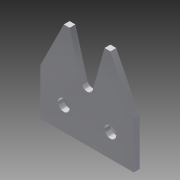
# Autodesk Inventor part: pickup arm tab
Saved by Autodesk Inventor 2015 (Build 190159000, 159)
## iProperties
Created: 2015-01-20
Part Number: pickup arm tab
Material: Aluminum 6061
Document SubType Name: Modeling
Designer: Jarod
Density: 2.7 g/cm^3
Appearance: Aluminum - Flat
Author: Jarod
Autodesk Inventor part; units mm, degrees
ref_plane "YZ Plane" through (0, 0, 0) normal (1, 0, 0) x (0, 1, 0)
ref_plane "XZ Plane" through (0, 0, 0) normal (0, 1, 0) x (-1, 0, 0)
ref_plane "XY Plane" through (0, 0, 0) normal (0, 0, 1) x (1, 0, 0)
sketch "Sketch1" plane through (0, 0, 0) normal (0, 0, 1) x (1, 0, 0)
  line L0 (0, 0) -> (50.8, 0)
  line L1 (50.8, 0) -> (50.8, 50.8)
  line L2 (50.8, 50.8) -> (0, 50.8)
  line L3 (0, 50.8) -> (0, 0)
  dimension "d0" = 50.8
  dimension "d1" = 50.8
  constraints: 8 end point, 2 parallel, 1 horizontal, 1 perpendicular
  measures "d0" distance of L2.end L1.end
  measures "d1" distance of L1.end L0.end
extrude "Extrusion1" add sketch "Sketch1" along normal blind 3.175
sketch "Sketch2" plane through (0, 0, 3.175) normal (0, 0, 1) x (1, 0, 0)
  line L0 (0, 0) -> (50.8, 0) projected
  line L1 (50.8, 0) -> (50.8, 50.8) projected
  line L2 (50.8, 50.8) -> (0, 50.8) projected
  line L3 (0, 50.8) -> (0, 0) projected
  point P0 (12.7, 12.7)
  point P1 (38.1, 12.7)
  dimension "d4" = 12.7
  dimension "d5" = 12.7
  dimension "d6" = 12.7
  dimension "d7" = 12.7
  measures "d4" distance from line of L0 point (12.7, 12.7)
  measures "d5" distance from line of L3 point (12.7, 12.7)
  measures "d6" distance from line of L0 point (38.1, 12.7)
  measures "d7" distance from line of L1 point (38.1, 12.7)
hole "Hole1" at (12.7, 12.7, 3.175) at (38.1, 12.7, 3.175) direction (0, 0, -1) diameter 6.35 end through all
sketch "Sketch3" plane through (0, 0, 0) normal (0, 0, -1) x (-1, 0, 0)
  line L0 (0, 0) -> (-50.8, 0) projected
  line L1 (-50.8, 0) -> (-50.8, 50.8) projected
  line L2 (-50.8, 0) -> (-50.8, 50.8) projected
  line L3 (-50.8, 25.4) -> (-38.1, 50.8)
  line L4 (-50.8, 50.8) -> (0, 50.8) construction
  line L5 (-38.1, 50.8) -> (-12.7, 50.8) construction
  line L6 (-12.7, 50.8) -> (0, 25.4)
  line L7 (0, 50.8) -> (0, 0) projected
  line L8 (-38.1, 50.8) -> (-50.8, 50.8)
  line L9 (-50.8, 50.8) -> (-50.8, 25.4)
  line L10 (-12.7, 50.8) -> (0, 50.8)
  line L11 (0, 50.8) -> (0, 25.4)
  dimension "d19" = 25.4
  dimension "d20" = 25.4
  dimension "d21" = 25.4
  dimension "d22" = 12.7
  constraints: 14 end point, 2 collinear, 2 midpoint, 2 perpendicular, 2 point on line
  measures "d19" distance of L5.end L3.end
  measures "d20" distance from line of L0 L3.start
  measures "d21" distance from line of L0 L6.end
  measures "d22" distance from line of L1 L3.end
extrude "Extrusion2" cut sketch "Sketch3" against normal blind 25.4
sketch "Sketch4" plane through (0, 0, 0) normal (0, 0, -1) x (-1, 0, 0)
  line L0 (0, 25.4) -> (-12.7, 50.8) projected
  line L1 (-38.1, 50.8) -> (-12.7, 50.8) projected
  line L2 (-38.1, 50.8) -> (-50.8, 25.4) projected
  line L3 (-50.8, 0) -> (-50.8, 25.4) projected
  line L4 (0, 0) -> (-50.8, 0) projected
  line L5 (0, 25.4) -> (0, 0) projected
  circle A0 centre (-12.7, 12.7) radius 3.175 projected
  circle A1 centre (-38.1, 12.7) radius 3.175 projected
  circle A2 centre (-25.4, 28.575) radius 3.175 construction
  line L6 (-34.925, 50.8) -> (-28.4572, 27.7183)
  line L7 (-15.875, 50.8) -> (-22.3428, 27.7183)
  arc A3 (-28.4572, 27.7183) -> (-22.3428, 27.7183) centre (-25.4, 28.575) ccw
  line L8 (-34.925, 50.8) -> (-15.875, 50.8)
  line L9 (-38.1, 50.8) -> (-12.7, 50.8) projected
  dimension "d25" = 6.35
  dimension "d26" = 22.225
  dimension "d27" = 12.7
  dimension "d28" = 3.175
  dimension "d29" = 3.175
  constraints: 6 end point, 4 point on circle, 4 tangent, 2 centre point, 2 point on line, 1 collinear
  measures "d25" diameter of A2
  measures "d26" distance from line of A2.centre L1
  measures "d27" horizontal distance of L0.end A2.centre
  measures "d28" distance of L1.start L6.start
  measures "d29" distance of L0.end L7.start
extrude "Extrusion3" cut sketch "Sketch4" against normal blind 25.4 contours L7 A3 L6 L1
body "Solid1"
